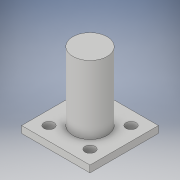
# Autodesk Inventor part: Laserhalter Mittelteil 29112018
Saved by Autodesk Inventor 2018.3 (Build 223284000, 284)
## iProperties
Created: 2018-11-29
Part Number: Laserhalter Mittelteil 29112018
Material: Generisch
Document SubType Name: Modeling
Designer: pgmadmin
Density: 1 g/cm^3
Appearance: Vorgabe
Author: pgmadmin
Autodesk Inventor part; units mm, degrees
ref_plane "YZ Plane" through (0, 0, 0) normal (1, 0, 0) x (0, 1, 0)
ref_plane "XZ Plane" through (0, 0, 0) normal (0, 1, 0) x (-1, 0, 0)
ref_plane "XY Plane" through (0, 0, 0) normal (0, 0, 1) x (1, 0, 0)
sketch "Skizze1" plane through (0, 0, 0) normal (0, 0, 1) x (1, 0, 0)
  line L0 (-10, -10) -> (10, -10)
  line L1 (10, -10) -> (10, 10)
  line L2 (10, 10) -> (-10, 10)
  line L3 (-10, 10) -> (-10, -10)
  line L4 (-10, -10) -> (10, 10) construction
  line L5 (10, -10) -> (-10, 10) construction
  point P0 (0, 0)
  dimension "d0" = 20
  dimension "d1" = 20
  constraints: 12 end point, 2 midpoint, 2 parallel, 1 horizontal, 1 perpendicular
  measures "d0" distance of L1.end L2.end
  measures "d1" distance of L0.end L1.end
extrude "Extrusion1" add sketch "Skizze1" along normal blind 2
sketch "Skizze2" plane through (0, 0, 2) normal (0, 0, 1) x (1, 0, 0)
  circle A0 centre (0, 0) radius 5
  dimension "d4" = 10
  constraints: 1 centre point, 1 coincident
  measures "d4" diameter of A0
extrude "Extrusion2" add sketch "Skizze2" along normal blind 20
sketch "Skizze3" plane through (0, 0, 2) normal (0, 0, 1) x (1, 0, 0)
  line L0 (10, 10) -> (-10, 10) projected
  line L1 (-10, 10) -> (-10, -10) projected
  line L2 (10, -10) -> (10, 10) projected
  line L3 (-10, -10) -> (10, -10) projected
  point P0 (0, 0)
  point P1 (-6, 6)
  point P2 (6, 6)
  point P3 (6, -6)
  point P4 (-6, -6)
  dimension "d7" = 4
  dimension "d8" = 4
  dimension "d9" = 4
  dimension "d10" = 4
  dimension "d11" = 4
  dimension "d12" = 4
  dimension "d13" = 4
  dimension "d14" = 4
  measures "d7" distance from line of L0 point (-6, 6)
  measures "d8" distance from line of L1 point (-6, 6)
  measures "d9" distance from line of L2 point (6, 6)
  measures "d10" distance from line of L0 point (6, 6)
  measures "d11" distance from line of L2 point (6, -6)
  measures "d12" distance from line of L3 point (6, -6)
  measures "d13" distance from line of L3 point (-6, -6)
  measures "d14" distance from line of L1 point (-6, -6)
hole "Bohrung1" at (-6, 6, 2) at (6, 6, 2) at (6, -6, 2) at (-6, -6, 2) direction (0, 0, -1) diameter 2.95 end through all
